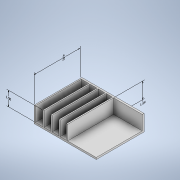
# Autodesk Inventor part: shelfForElectronicsV01
Saved by Autodesk Inventor 2021.2 (Build 252289000, 289)
## iProperties
Created: 2020-12-15
Part Number: shelfForElectronicsV01
Material: Generic
Document SubType Name: Modeling
Designer: robst
Density: 1 g/cm^3
Appearance: Default
Author: robst
Autodesk Inventor part; units mm, degrees
ref_plane "YZ Plane" through (0, 0, 0) normal (1, 0, 0) x (0, 1, 0)
ref_plane "XZ Plane" through (0, 0, 0) normal (0, 1, 0) x (-1, 0, 0)
ref_plane "XY Plane" through (0, 0, 0) normal (0, 0, 1) x (1, 0, 0)
sketch "Sketch2" plane through (0, 0, 0) normal (0, 1, 0) x (-1, 0, 0)
  line L0 (44.45, 63.5) -> (-44.45, 63.5)
  line L1 (-44.45, 63.5) -> (-44.45, -63.5)
  line L2 (-44.45, -63.5) -> (44.45, -63.5)
  line L3 (44.45, -63.5) -> (44.45, 63.5)
  line L4 (44.45, 63.5) -> (-44.45, -63.5) construction
  line L5 (-44.45, 63.5) -> (44.45, -63.5) construction
  point P0 (0, 0)
  dimension "d0" = 127
  dimension "d1" = 88.9
  constraints: 12 end point, 2 midpoint, 2 parallel, 1 horizontal, 1 perpendicular
  measures "d0" distance of L2.end L0.start
  measures "d1" distance of L1.end L2.end
extrude "Extrusion1" add sketch "Sketch2" against normal blind 4.7625
sketch "Sketch4" plane through (0, 0, 0) normal (0, 1, 0) x (1, 0, 0)
  line L0 (-44.45, -63.5) -> (-44.45, 63.5) projected
  line L1 (44.45, 63.5) -> (44.45, -63.5) projected
  line L2 (-44.45, 63.5) -> (44.45, 63.5)
  line L3 (44.45, 63.5) -> (44.45, 58.7375)
  line L4 (44.45, 58.7375) -> (-44.45, 58.7375)
  line L5 (-44.45, 58.7375) -> (-44.45, 63.5)
  point P0 (0, 0)
  point P1 (-44.45, 58.7375)
  dimension "d4" = 4.7625
  constraints: 8 end point, 2 parallel, 1 horizontal, 1 perpendicular, 1 point on line
  measures "d4" distance between parallel lines of L4 L2
extrude "Extrusion2" add sketch "Sketch4" along normal blind 38.1
sketch "Sketch5" plane through (0, 0, 0) normal (0, 1, 0) x (1, 0, 0)
  line L0 (44.45, -63.5) -> (-44.45, -63.5) projected
  line L1 (-44.45, 58.7375) -> (44.45, 58.7375) projected
  line L2 (-44.45, -63.5) -> (-41.275, -63.5)
  line L3 (-41.275, -63.5) -> (-41.275, 58.7375)
  line L4 (-44.45, 58.7375) -> (-44.45, -63.5)
  line L5 (44.45, 63.5) -> (44.45, -63.5) projected
  line L6 (44.45, -63.5) -> (41.275, -63.5)
  line L7 (41.275, -63.5) -> (41.275, 58.7375)
  line L8 (44.45, 58.7375) -> (44.45, -63.5)
  line L9 (-44.45, 58.7375) -> (-44.45, -63.5) projected
  line L10 (-44.45, -63.5) -> (-44.45, 63.5) projected
  line L11 (-44.45, 58.7375) -> (-44.45, 63.5)
  line L12 (-44.45, 63.5) -> (-41.275, 63.5)
  line L13 (-44.45, 63.5) -> (44.45, 63.5) projected
  line L14 (-41.275, 58.7375) -> (-41.275, 63.5)
  line L15 (44.45, 58.7375) -> (-44.45, 58.7375) projected
  line L16 (44.45, 58.7375) -> (44.45, 63.5)
  line L17 (41.275, 63.5) -> (41.275, 58.7375)
  point P0 (0, 0)
  point P1 (41.275, 58.7375)
  point P2 (-44.45, 58.7375)
  point P3 (41.275, 58.7375)
  dimension "d7" = 3.175
  dimension "d8" = 3.175
  constraints: 22 end point, 3 parallel, 3 perpendicular, 3 point on line, 2 horizontal, 1 collinear, 1 vertical
  measures "d7" distance between parallel lines of L3 L4
  measures "d8" distance between parallel lines of L5 L7
extrude "Extrusion3" add sketch "Sketch5" along normal blind 38.1 contours L0 L7 L1 L5 | L1 L17 L13 L5 | L0 L4 L1 L3 | L1 L10 L12 L14
sketch "Sketch6" plane through (0, 0, 0) normal (0, 1, 0) x (1, 0, 0)
  line L0 (-41.275, -63.5) -> (41.275, -63.5) projected
  line L1 (-41.275, 58.7375) -> (41.275, 58.7375) projected
  line L2 (-21.4312, -63.5) -> (-18.2562, -63.5)
  line L3 (-18.2562, -63.5) -> (-18.2563, 58.7375)
  line L4 (-18.2563, 58.7375) -> (-21.4313, 58.7375)
  line L5 (-21.4313, 58.7375) -> (-21.4312, -63.5)
  line L6 (0, -63.5) -> (3.175, -63.5)
  line L7 (3.175, -63.5) -> (3.175, 58.7375)
  line L8 (3.175, 58.7375) -> (0, 58.7375)
  line L9 (0, 58.7375) -> (0, -63.5)
  line L10 (21.4313, -63.5) -> (24.6063, -63.5)
  line L11 (24.6063, -63.5) -> (24.6063, 58.7375)
  line L12 (24.6063, 58.7375) -> (21.4312, 58.7375)
  line L13 (21.4312, 58.7375) -> (21.4313, -63.5)
  line L14 (-39.6875, -63.5) -> (-39.6875, 58.7375) projected
  line L15 (39.6875, 58.7375) -> (39.6875, -63.5) projected
  point P0 (0, 0)
  point P1 (21.4313, -63.5)
  point P2 (24.6063, -63.5)
  point P3 (24.6063, 58.7375)
  point P4 (0, 58.7375)
  point P5 (0, -63.5)
  point P6 (3.175, -63.5)
  dimension "d11" = 3.175
  dimension "d12" = 3.175
  dimension "d13" = 3.175
  dimension "d14" = 18.2563
  dimension "d15" = 18.2563
  dimension "d16" = 18.2563
  dimension "d17" = 15.0813
  constraints: 24 end point, 6 parallel, 6 point on line, 3 horizontal, 3 perpendicular
  measures "d11" distance between parallel lines of L3 L5
  measures "d12" distance between parallel lines of L7 L9
  measures "d13" distance between parallel lines of L11 L13
  measures "d14" distance between parallel lines of L9 L3
  measures "d15" distance between parallel lines of L13 L7
  measures "d16" distance between parallel lines of L5 L14
  measures "d17" distance between parallel lines of L11 L15
extrude "Extrusion4" add sketch "Sketch6" along normal blind 38.1 contours L5 L1 L3 L0 | L9 L1 L7 L0 | L13 L1 L11 L0
sketch "Sketch9" plane through (44.45, -4.7625, 63.5) normal (1, 0, 0) x (0, 0, -1)
  line L0 (0, 0) -> (0, 42.8625) projected
  line L1 (127, 0) -> (127, 42.8625) projected
  line L2 (0, 0) -> (127, 0)
  line L3 (127, 0) -> (127, 4.7625)
  line L4 (127, 4.7625) -> (0, 4.7625)
  line L5 (0, 4.7625) -> (0, 0)
  point P0 (63.5, 4.7625)
  dimension "d37" = 4.7625
  constraints: 8 end point, 2 parallel, 1 horizontal, 1 perpendicular, 1 point on line
  measures "d37" distance between parallel lines of L4 L2
extrude "Extrusion5" add sketch "Sketch9" along normal blind 76.2
sketch "Sketch10" plane through (44.45, 38.1, 63.5) normal (1, 0, 0) x (0, 0, -1)
  line L0 (127, -38.1) -> (127, 0) projected
  line L1 (122.2375, 0) -> (0, 0) projected
  line L2 (127, -38.1) -> (122.2375, -38.1)
  line L3 (122.2375, -38.1) -> (122.2375, 0)
  line L4 (122.2375, 0) -> (127, 0)
  line L5 (127, 0) -> (127, -38.1)
  point P0 (63.5, -38.1)
  constraints: 8 end point, 2 parallel, 1 horizontal, 1 perpendicular
extrude "Extrusion6" add sketch "Sketch10" along normal blind 76.2
equation "\"d0\" = depth"
equation "\"d1\" = width"
equation "\"d2\" = baseThickness"
equation "\"d4\" = backThickness"
equation "\"d5\" = backHeight"
equation "\"d7\" = edgeThickness"
equation "\"d8\" = edgeThickness"
equation "\"d9\" = edgeHeight"
equation "\"d11\" = dividerThickness"
equation "\"d12\" = dividerThickness"
equation "\"d13\" = dividerThickness"
equation "\"d14\" = dividerGap"
equation "\"d15\" = dividerGap"
equation "\"d16\" = dividerGap"
equation "\"d19\" = dividerHeight"
equation "\"d37\" = baseThickness"
equation "\"d38\" = waterShelfWidth"
equation "\"d40\" = waterShelfWidth"
equation "\"baseThickness\" = 4.7625"
equation "\"width\" = 88.9"
equation "\"depth\" = 127"
equation "\"backHeight\" = 38.1"
equation "\"backThickness\" = 4.7625"
equation "\"edgeThickness\" = 3.175"
equation "\"edgeHeight\" = 38.1"
equation "\"dividerThickness\" = 3.175"
equation "\"dividerHeight\" = 38.1"
equation "\"waterShelfWidth\" = 76.2"
equation "\"dividerGap\" = 18.25625"
body "Solid1"
